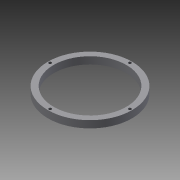
# Autodesk Inventor part: PMT Cap
Saved by Autodesk Inventor 2015 (Build 190159000, 159)
## iProperties
Created: 2014-07-10
Part Number: PMT Cap
Material: Generic
Document SubType Name: Modeling
Designer: I Rabey
Density: 1 g/cm^3
Appearance: Default
Author: I Rabey
Autodesk Inventor part; units mm, degrees
ref_plane "YZ Plane" through (0, 0, 0) normal (1, 0, 0) x (0, 1, 0)
ref_plane "XZ Plane" through (0, 0, 0) normal (0, 1, 0) x (-1, 0, 0)
ref_plane "XY Plane" through (0, 0, 0) normal (0, 0, 1) x (1, 0, 0)
sketch "Sketch1" plane through (0, 0, 0) normal (0, 1, 0) x (-1, 0, 0)
  circle A0 centre (0, 0) radius 25.5
  circle A1 centre (0, 0) radius 29.5
  dimension "d0" = 51
  dimension "d1" = 59
  constraints: 2 centre point, 2 coincident
  measures "d0" diameter of A0
  measures "d1" diameter of A1
extrude "Extrusion1" add sketch "Sketch1" along normal blind 5
sketch "Sketch2" plane through (0, 5, 0) normal (0, 1, 0) x (1, 0, 0)
  circle A0 centre (0, -28) radius 1
  point P0 (0, 0)
  dimension "d4" = 2
  dimension "d5" = 28
  constraints: 1 centre point
  measures "d4" diameter of A0
  measures "d5" distance of point (0, 0) A0.centre
sketch "Sketch3" plane through (0, 5, 0) normal (0, 1, 0) x (1, 0, 0)
  circle A0 centre (-28, 0) radius 1
  point P0 (0, 0)
  dimension "d6" = 2
  dimension "d7" = 28
  constraints: 1 centre point
  measures "d6" diameter of A0
  measures "d7" distance of point (0, 0) A0.centre
sketch "Sketch4" plane through (0, 5, 0) normal (0, 1, 0) x (1, 0, 0)
  circle A0 centre (0, 28) radius 1
  point P0 (0, 0)
  dimension "d8" = 2
  dimension "d9" = 28
  constraints: 1 centre point
  measures "d8" diameter of A0
  measures "d9" distance of A0.centre point (0, 0)
sketch "Sketch5" plane through (0, 5, 0) normal (0, 1, 0) x (1, 0, 0)
  circle A0 centre (28, 0) radius 1
  point P0 (0, 0)
  dimension "d10" = 2
  dimension "d11" = 28
  constraints: 1 centre point
  measures "d10" diameter of A0
  measures "d11" distance of point (0, 0) A0.centre
hole "Hole1" at (0, 5, 28) direction (0, -1, 0) diameter 2 depth 3 tip angle 118
hole "Hole2" at (-28, 5, 0) direction (0, -1, 0) diameter 2 depth 3 tip angle 118
hole "Hole3" at (0, 5, -28) direction (0, -1, 0) diameter 2 depth 3 tip angle 118
hole "Hole4" at (28, 5, 0) direction (0, -1, 0) diameter 2 depth 3 tip angle 118
thread "Thread1" size "M2x0.4" class "6H" standard "ANSI Metric M Profile" full length
thread "Thread2" size "M2x0.4" class "6H" standard "ANSI Metric M Profile" full length
thread "Thread3" size "M2x0.4" class "6H" standard "ANSI Metric M Profile" full length
thread "Thread4" size "M2x0.4" class "6H" standard "ANSI Metric M Profile" full length
body "Solid1"
